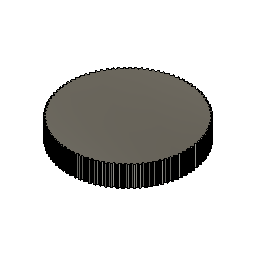
gear_91z (Autodesk Fusion 360 design; units mm, degrees)
Autodesk Fusion 360 part; units mm, degrees
sketch "Sketch1" plane through (0, 0, 0) normal (0, 0, 1) x (1, 0, 0) in component "gt2 pulley"
  circle A0 centre (0, 0) radius 28.9662 construction
  circle A1 centre (0, 0) radius 27.9622 construction
  line L0 (0, 0) -> (0, 28.9662) construction
  line L1 (0, 0) -> (0.9998, 28.9489) construction
  line L2 (0, 0) -> (1.4044, 28.9321) construction
  circle A2 centre (0, 0) radius 28.7122 construction
  arc A3 (0.3973, 28.5764) -> (0.4758, 28.2779) centre (1.3921, 28.6784) ccw
  circle A4 centre (0, 0) radius 28.5622 construction
  arc A5 (0.2493, 28.7111) -> (0, 28.7122) centre (0, 0) ccw
  arc A6 (0.3973, 28.5764) -> (0.2493, 28.7111) centre (0.2481, 28.5611) ccw
  arc A7 (0.4758, 28.2779) -> (0.9651, 27.9455) centre (0.9843, 28.5002) ccw
  arc A8 (0, 28.7122) -> (-0.2493, 28.7111) centre (0, 0) ccw
  arc A9 (-0.2493, 28.7111) -> (-0.3973, 28.5764) centre (-0.2481, 28.5611) ccw
  arc A10 (-0.4758, 28.2779) -> (-0.3973, 28.5764) centre (-1.3921, 28.6784) ccw
  arc A11 (-0.965, 27.9455) -> (-0.4758, 28.2779) centre (-0.9843, 28.5002) ccw
  arc A12 (0.9651, 27.9455) -> (-0.9651, 27.9455) centre (0, 0) ccw
  point P0 (1.3921, 28.6784)
  point P1 (0, 28.7122)
  dimension "d18" = 57.9324
  dimension "d19" = 1.978
  dimension "d22" = 1.004
  dimension "d24" = 0.75
  dimension "d26" = 1
  dimension "d27" = 0.15
  dimension "d28" = 0.15
  dimension "d47" = 0.555
  dimension "d52" = 3.812
  constraint coincident A0.centre A1.centre
  constraint coincident A0 L0.end
  constraint vertical L0
  constraint coincident A0 L1.end
  constraint coincident A0 L2.end
  constraint concentric A1 A2
  constraint coincident A1 A7.end
  constraint coincident L1 A7.end
  constraint coincident A2 P0
  constraint coincident L2 P0
  constraint coincident P0 A3.centre
  constraint coincident A2 P1
  constraint coincident L0 P1
  constraint concentric A2 A4
  constraint coincident P1 A5.end
  constraint coincident A4 A6.centre
  constraint coincident A3.start A6.start
  constraint tangent A3 A6
  constraint tangent A3 A7
  constraint symmetric L0 A7.end A12.end
  constraint symmetric L0 A3.start A9.end
  constraint symmetric L0 A3.end A10.start
  constraint symmetric L0 A3 A10
  constraint symmetric L0 A5.start A8.end
  constraint symmetric L0 P1 A5.end
  constraint symmetric L0 A5 A8
  constraint symmetric L0 A6 A9
  constraint symmetric L0 A7 A11
  constraint coincident A1 A11.start
  constraint tangent A1 A7
  constraint coincident L1 A7.centre
  measures "d18" diameter of A0
  measures "d19" angle of L0 L1
  measures "d22" distance of A0 A1
  measures "d24" distance of A1 A2
  measures "d26" radius of A3
  measures "d27" distance of A2 A4
  measures "d28" radius of A6
  measures "d47" radius of A7
extrude "Extrude1" add sketch "Sketch1" along normal blind 10 makes body 1
pattern_circular "C-Pattern1" count 91 over 360 about axis through (0, 0, 1.75) along (0, 0, 1) of bodies 1 makes body 2 at (-2.6773, 27.8337, 6.6667) makes body 3 at (-3.9552, 27.6811, 6.6667) makes body 4 at (-6.2744, 27.2492, 6.6667) makes body 5 at (-6.8999, 27.0975, 3.3333) makes body 6 at (-8.7529, 26.5569, 3.3333) makes body 7 at (-11.3536, 25.5535, 6.6667) makes body 8 at (-13.6546, 24.4015, 6.6667) makes body 9 at (-15.3056, 23.4014, 6.6667) makes body 10 at (-16.8836, 22.2896, 6.6667) makes body 11 at (-17.726, 21.6257, 6.6667) makes body 12 at (-18.7024, 20.7871, 3.3333) makes body 13 at (-20.0919, 19.4473, 3.3333) makes body 14 at (-22.3219, 16.841, 6.6667) makes body 15 at (-23.3128, 15.4402, 6.6667) makes body 16 at (-23.662, 14.8995, 3.3333) makes body 17 at (-24.6335, 13.2315, 3.3333) makes body 18 at (-25.4877, 11.5005, 3.3333) makes body 19 at (-26.2204, 9.7147, 3.3333) makes body 20 at (-26.8282, 7.8826, 3.3333) makes body 21 at (-27.3081, 6.0129, 3.3333) makes body 22 at (-27.771, 3.264, 6.6667) makes body 23 at (-27.9301, 1.3403, 6.6667) makes body 24 at (-27.9609, 0.2682, 3.3333) makes body 25 at (-27.9128, -1.6615, 3.3333) makes body 26 at (-27.6087, -4.4324, 6.6667) makes body 27 at (-27.4184, -5.488, 3.3333) makes body 28 at (-26.5401, -8.8037, 6.6667) makes body 29 at (-25.8695, -10.6138, 6.6667) makes body 30 at (-25.0756, -12.3733, 6.6667) makes body 31 at (-24.4797, -13.514, 6.6667) makes body 32 at (-23.1337, -15.7072, 6.6667) makes body 33 at (-22.8899, -16.0604, 6.6667) makes body 34 at (-21.7273, -17.6013, 3.3333) makes body 35 at (-20.4612, -19.0584, 3.3333) makes body 36 at (-17.9738, -21.4202, 6.6667) makes body 37 at (-16.9691, -22.2246, 6.6667) makes body 38 at (-16.1043, -22.859, 3.3333) makes body 39 at (-13.1843, -24.6588, 6.6667) makes body 40 at (-12.8044, -24.8583, 3.3333) makes body 41 at (-11.0589, -25.6824, 3.3333) makes body 42 at (-8.4468, -26.6559, 6.6667) makes body 43 at (-6.17, -27.273, 6.6667) makes body 44 at (-5.5406, -27.4078, 3.3333) makes body 45 at (-3.6365, -27.7247, 3.3333) makes body 46 at (-1.7151, -27.9096, 3.3333) makes body 47 at (0.2145, -27.9614, 3.3333) makes body 48 at (2.9974, -27.8011, 6.6667) makes body 49 at (5.5405, -27.4078, 6.6667) makes body 50 at (7.4182, -26.9603, 6.6667) makes body 51 at (7.8311, -26.8432, 3.3333) makes body 52 at (9.6643, -26.239, 3.3333) makes body 53 at (12.8043, -24.8583, 6.6667) makes body 54 at (14.4887, -23.9157, 6.6667) makes body 55 at (15.5739, -23.2237, 6.6667) makes body 56 at (16.4531, -22.6093, 6.6667) makes body 57 at (17.9737, -21.4203, 3.3333) makes body 58 at (20.4611, -19.0585, 6.6667) makes body 59 at (20.7512, -18.7422, 3.3333) makes body 60 at (22.3863, -16.7552, 6.6667) makes body 61 at (23.6046, -14.9902, 6.6667) makes body 62 at (24.5826, -13.326, 6.6667) makes body 63 at (25.7035, -11.0097, 6.6667) makes body 64 at (26.1069, -10.0158, 6.6667) makes body 65 at (26.7977, -7.9855, 6.6667) makes body 66 at (27.2848, -6.1176, 6.6667) makes body 67 at (27.6418, -4.2206, 6.6667) makes body 68 at (27.9128, -1.6617, 6.6667) makes body 69 at (27.9597, -0.3755, 6.6667) makes body 70 at (27.9535, 0.6971, 3.3333) makes body 71 at (27.6578, 4.1144, 6.6667) makes body 72 at (27.5914, 4.5384, 6.6667) makes body 73 at (26.8282, 7.8824, 6.6667) makes body 74 at (26.4371, 9.1086, 6.6667) makes body 75 at (25.4878, 11.5004, 6.6667) makes body 76 at (24.6336, 13.2314, 6.6667) makes body 77 at (24.4276, 13.6079, 6.6667) makes body 78 at (23.4306, 15.2608, 3.3333) makes body 79 at (22.3219, 16.8409, 3.3333) makes body 80 at (20.092, 19.4472, 6.6667) makes body 81 at (19.1759, 20.3512, 6.6667) makes body 82 at (17.3923, 21.8951, 6.6667) makes body 83 at (16.8837, 22.2896, 3.3333) makes body 84 at (14.5805, 23.8599, 6.6667) makes body 85 at (12.3254, 25.0992, 6.6667) makes body 86 at (10.5644, 25.8897, 6.6667) makes body 87 at (10.1658, 26.0488, 3.3333) makes body 88 at (6.9, 27.0975, 6.6667) makes body 89 at (6.4833, 27.2002, 3.3333) makes body 90 at (3.7429, 27.7106, 6.6667) makes body 91 at (1.1796, 27.9373, 6.6667)
sketch "Sketch2" plane through (0, 0, 10) normal (0, 0, 1) x (-1, 0, 0)
  arc A0 (-10.0445, -26.7559) -> (-9.9508, -26.9327) centre (-9.8989, -26.792) ccw
  arc A1 (-9.9508, -26.9327) -> (-9.4816, -27.1015) centre (0, 0) ccw
  arc A2 (-9.4816, -27.1015) -> (-9.2968, -27.0248) centre (-9.432, -26.9599) ccw
  arc A3 (-9.1219, -26.7705) -> (-9.2968, -27.0248) centre (-8.3952, -27.4574) ccw
  arc A4 (-8.5491, -26.6233) -> (-9.1219, -26.7705) centre (-8.7186, -27.1517) ccw
  arc A5 (-10.3653, -25.9701) -> (-8.5491, -26.6233) centre (0, 0) ccw
  arc A6 (-10.0173, -26.4485) -> (-10.3653, -25.9701) centre (-10.5711, -26.4855) ccw
  arc A7 (-10.0445, -26.7559) -> (-10.0173, -26.4485) centre (-11.0151, -26.5153) ccw
  circle A8 centre (0, 0) radius 27.9622
  constraint concentric A1 A8
extrude "Extrude2" add sketch "Sketch2" against normal blind 10 contours A5 A8 bodies 1 2 3 4 5 6 7 8 9 10 11 12 13 14 15 16 17 18 19 20 21 22 23 24 25 26 27 28 29 30 31 32 33 34 35 36 37 38 39 40 41 42 43 44 45 46 47 48 49 50 51 52 53 54 55 56 57 58 59 60 61 62 63 64 65 66 67 68 69 70 71 72 73 74 75 76 77 78 79 80 81 82 83 84 85 86 87 88 89 90 91
extrude "Extrude4" [suppressed] in component "gt2 pulley"
pattern_circular "C-Pattern7" [suppressed] in component "gt2 pulley"
extrude "Extrude3" [suppressed] in component "gt2 pulley"
pattern_circular "C-Pattern6" [suppressed] in component "gt2 pulley"
extrude "Extrude2'" [suppressed] in component "gt2 pulley"
pattern_circular "C-Pattern5" [suppressed] in component "gt2 pulley"
extrude "Extrude1'" [suppressed] in component "gt2 pulley"
pattern_circular "C-Pattern4" [suppressed] in component "gt2 pulley"
pattern_circular "C-Pattern3" [suppressed] in component "gt2 pulley"
pattern_circular "C-Pattern2" [suppressed] in component "gt2 pulley"
pattern_circular "C-Pattern1'" [suppressed] in component "gt2 pulley"
copy_body "Body->Comp1" [suppressed] in component "Component"
copy_body "Body->Comp2" [suppressed] in component "Component'"
copy_body "Body->Comp3" [suppressed] in component "Component''"
copy_body "Body->Comp4" [suppressed] in component "Component'''"
copy_body "Body->Comp5" [suppressed] in component "Component''''"
copy_body "Body->Comp6" [suppressed] in component "Component'''''"
copy_body "Body->Comp7" [suppressed] in component "Component''''''"
copy_body "Body->Comp8" [suppressed] in component "Component'''''''"
copy_body "Body->Comp9" [suppressed] in component "Component''''''''"
copy_body "Body->Comp10" [suppressed] in component "Component'''''''''"
copy_body "Body->Comp11" [suppressed] in component "Component''''''''''"
copy_body "Body->Comp12" [suppressed] in component "Component'''''''''''"
copy_body "Body->Comp13" [suppressed] in component "Component''''''''''''"
copy_body "Body->Comp14" [suppressed] in component "Component'''''''''''''"
copy_body "Body->Comp15" [suppressed] in component "Component''''''''''''''"
copy_body "Body->Comp16" [suppressed] in component "Component'''''''''''''''"
copy_body "Body->Comp17" [suppressed] in component "Component''''''''''''''''"
copy_body "Body->Comp18" [suppressed] in component "Component'''''''''''''''''"
copy_body "Body->Comp19" [suppressed] in component "Component''''''''''''''''''"
copy_body "Body->Comp20" [suppressed] in component "Component'''''''''''''''''''"
component "gt2 pulley" placed x (1, 0, 0) y (0, 1, 0) z (0, 0, 1) at (0, 0, 0)
equation "NumTeeth = 91" comment "min 20"
equation "ToothPitch = 2 mm"
equation "PullyDia = NumTeeth * ToothPitch / PI"
equation "ToothAng = ( ( 360 / NumTeeth ) * 1 deg )"
equation "TransOffsetAngle = ToothAng * 0.2"
equation "Sholulder_Radius = 0.15 mm"
equation "Root_Radius = 0.555 mm"
equation "TransRadius = 1 mm"
equation "ToolHeight = 0.75 mm"
equation "PLD = 0.254 mm"
equation "d18 = PullyDia"
equation "d19 = ToothAng / 2"
equation "d22 = PLD + ToolHeight"
equation "d24 = ToolHeight"
equation "d26 = TransRadius"
equation "d27 = Sholulder_Radius"
equation "d31 = NumTeeth"
equation "d33 = NumTeeth"
equation "d35 = NumTeeth"
equation "d37 = NumTeeth"
equation "d41 = NumTeeth"
equation "d45 = NumTeeth"
equation "d47 = Root_Radius"
equation "d50 = NumTeeth"
